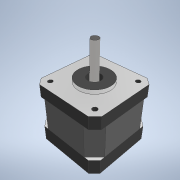
# Autodesk Inventor part: Nema-17
Saved by Autodesk Inventor 2021.1 (Build 251245010, 245A)
## iProperties
Created: 2022-01-16
Part Number: Nema-17
Material: Типовые
Document SubType Name: Modeling
Designer: Andrew
Density: 1 g/cm^3
Appearance: По умолчанию
Author: Andrew
Autodesk Inventor part; units mm, degrees
ref_plane "YZ Plane" through (0, 0, 0) normal (1, 0, 0) x (0, 1, 0)
ref_plane "XZ Plane" through (0, 0, 0) normal (0, 1, 0) x (-1, 0, 0)
ref_plane "XY Plane" through (0, 0, 0) normal (0, 0, 1) x (1, 0, 0)
sketch "Эскиз1" plane through (0, 0, 0) normal (0, 1, 0) x (-1, 0, 0)
  line L0 (9, 9) -> (-33, 9)
  line L1 (-33, 9) -> (-33, -33)
  line L2 (-33, -33) -> (9, -33)
  line L3 (9, -33) -> (9, 9)
  line L4 (9, -29) -> (5, -33)
  line L5 (9, 9) -> (-33, -33) construction
  line L6 (9, -33) -> (-33, 9) construction
  line L7 (5, 9) -> (9, 5)
  line L8 (-33, 5) -> (-29, 9)
  line L9 (-33, -29) -> (-29, -33)
  line L10 (13.5, -3.75) -> (9, -3.75)
  line L11 (9, -20.25) -> (13.5, -20.25)
  line L12 (13.5, -20.25) -> (13.5, -3.75)
  point P0 (0, 0)
  dimension "d0" = 42
  dimension "d1" = 42
  dimension "d2" = 4
  dimension "d3" = 4
  dimension "d17" = 12.75
  dimension "d18" = 16.5
  dimension "d19" = 4.5
  constraints: 26 end point, 10 point on line, 6 perpendicular, 2 parallel, 1 horizontal
  measures "d0" distance of L2.end L1.end
  measures "d1" distance of L1.end L0.end
  measures "d2" distance of L2.end L4.start
  measures "d3" distance of L4.end L2.end
  measures "d17" distance between parallel lines of L0 L10
  measures "d18" distance of L11.end L10.start
  measures "d19" distance of L11.start L11.end
extrude "Выдавливание1" add sketch "Эскиз1" along normal blind 9.5 contours L7 L3 L4 L2 L9 L1 L8 L0 | L10 L12 L11 L3
sketch "Эскиз2" plane through (0, 0, 0) normal (0, -1, 0) x (1, 0, 0)
  line L0 (-9, -33) -> (33, -33)
  line L1 (33, -33) -> (33, 9)
  line L2 (33, 9) -> (-9, 9)
  line L3 (-9, 9) -> (-9, -33)
  line L4 (-9, -33) -> (33, 9) construction
  line L5 (33, -33) -> (-9, 9) construction
  circle A0 centre (12, -12) radius 4.5
  circle A1 centre (-3.5, -27.5) radius 3.25
  circle A2 centre (-3.5, 3.5) radius 3.25
  circle A3 centre (27.5, 3.5) radius 3.25
  circle A4 centre (27.5, -27.5) radius 3.25
  line L6 (33, 5) -> (33, -29) projected
  line L7 (-5, 9) -> (29, 9) projected
  line L8 (29, -33) -> (-5, -33) projected
  line L9 (-9, -3.75) -> (-9, 5) projected
  point P0 (0, 0)
  dimension "d22" = 9
  dimension "d23" = 6.5
  dimension "d25" = 5.5
  dimension "d28" = 360
  constraints: 12 end point, 5 centre point, 4 collinear, 3 coincident, 2 parallel, 1 horizontal, 1 midpoint, 1 perpendicular, 1 point on line, 11 other
  measures "d22" diameter of A0
  measures "d23" diameter of A1
  measures "d25" distance from line of L0 A1.centre
extrude "Выдавливание2" cut sketch "Эскиз2" against normal blind 5 contours A0 | A1 | A2 | A3 | A4
sketch "Эскиз3" plane through (0, 9.5, 0) normal (0, 1, 0) x (1, 0, 0)
  line L0 (-13.5, 3.75) -> (-9, 3.75) projected
  line L1 (-13.5, 3.75) -> (-9, 3.75)
  line L2 (-9, 3.75) -> (-9, 20.25)
  line L3 (-9, 20.25) -> (-13.5, 20.25)
  line L4 (-13.5, 20.25) -> (-13.5, 3.75)
  point P0 (0, 0)
  constraints: 8 end point, 2 parallel, 1 horizontal, 1 perpendicular
extrude "Выдавливание3" cut sketch "Эскиз3" against normal blind 6
sketch "Эскиз4" plane through (-9, 0, -29) normal (-1, 0, 0) x (0, 0, 1)
  line L0 (8.75, 3.5) -> (25.25, 3.5) projected
  line L1 (8.75, 3.5) -> (25.25, 3.5)
  line L2 (25.25, 3.5) -> (25.25, 9.5)
  line L3 (25.25, 9.5) -> (8.75, 9.5)
  line L4 (8.75, 9.5) -> (8.75, 3.5)
  point P0 (29, 0)
  dimension "d34" = 16.5
  dimension "d35" = 6
  constraints: 8 end point, 2 parallel, 1 horizontal, 1 perpendicular
  measures "d34" distance of L3.end L2.end
  measures "d35" distance of L2.end L1.end
extrude "Выдавливание4" add sketch "Эскиз4" along normal blind 6 separate body
sketch "Эскиз5" plane through (-15, 0, -29) normal (-1, 0, 0) x (0, 0, 1)
  line L0 (25.25, 9.5) -> (8.75, 9.5) projected
  line L1 (25.25, 3.5) -> (8.75, 3.5) projected
  line L2 (8.75, 9.5) -> (25.25, 9.5)
  line L3 (25.25, 9.5) -> (25.25, 3.5)
  line L4 (25.25, 3.5) -> (8.75, 3.5)
  line L5 (8.75, 3.5) -> (8.75, 9.5)
  line L6 (9.75, 8.5) -> (12.75, 8.5)
  line L7 (24.25, 8.5) -> (24.25, 4.5)
  line L8 (24.25, 4.5) -> (9.75, 4.5)
  line L9 (9.75, 4.5) -> (9.75, 8.5)
  line L10 (12.75, 8.5) -> (12.75, 9.5)
  line L11 (21.25, 8.5) -> (21.25, 9.5)
  line L12 (0, 9.5) -> (34, 9.5) projected
  line L13 (21.25, 8.5) -> (24.25, 8.5)
  point P0 (29, 0)
  dimension "d38" = 1
  dimension "d39" = 4
  dimension "d40" = 4
  constraints: 22 end point, 5 parallel, 5 perpendicular, 3 point on line, 1 horizontal, 2 other
  measures "d38" distance between parallel lines of L5 L9
  measures "d39" distance between parallel lines of L10 L5
  measures "d40" distance between parallel lines of L11 L3
extrude "Выдавливание5" cut sketch "Эскиз5" against normal blind 6 contours L11 L13 L7 L8 L9 L6 L10 L0 bodies 2
sketch "Эскиз6" plane through (-9, 0, -29) normal (-1, 0, 0) x (0, 0, 1)
  line L0 (11.75, 7) -> (12.25, 7)
  line L1 (12.25, 7) -> (12.25, 6.5)
  line L2 (12.25, 6.5) -> (11.75, 6.5)
  line L3 (11.75, 6.5) -> (11.75, 7)
  line L4 (13.75, 7) -> (14.25, 7)
  line L5 (14.25, 7) -> (14.25, 6.5)
  line L6 (14.25, 6.5) -> (13.75, 6.5)
  line L7 (13.75, 6.5) -> (13.75, 7)
  line L8 (15.75, 7) -> (16.25, 7)
  line L9 (16.25, 7) -> (16.25, 6.5)
  line L10 (16.25, 6.5) -> (15.75, 6.5)
  line L11 (15.75, 6.5) -> (15.75, 7)
  line L12 (17.75, 7) -> (18.25, 7)
  line L13 (18.25, 7) -> (18.25, 6.5)
  line L14 (18.25, 6.5) -> (17.75, 6.5)
  line L15 (17.75, 6.5) -> (17.75, 7)
  line L16 (19.75, 7) -> (20.25, 7)
  line L17 (20.25, 7) -> (20.25, 6.5)
  line L18 (20.25, 6.5) -> (19.75, 6.5)
  line L19 (19.75, 6.5) -> (19.75, 7)
  line L20 (21.75, 7) -> (22.25, 7)
  line L21 (22.25, 7) -> (22.25, 6.5)
  line L22 (22.25, 6.5) -> (21.75, 6.5)
  line L23 (21.75, 6.5) -> (21.75, 7)
  line L24 (8.75, 0) -> (8.75, 3.5) projected
  point P0 (29, 0)
  dimension "d43" = 0.5
  dimension "d44" = 0.5
  dimension "d47" = 2
  dimension "d52" = 3
  constraints: 48 end point, 2 horizontal, 2 parallel, 1 collinear, 1 perpendicular, 39 other
  measures "d43" distance of L1.end L2.end
  measures "d44" distance of L0.end L1.end
  measures "d47" distance of L0.start L4.start
  measures "d52" distance between parallel lines of L24 L3
extrude "Выдавливание6" add sketch "Эскиз6" along normal blind 5 separate body
sketch "Эскиз7" plane through (0, 9.5, 0) normal (0, 1, 0) x (1, 0, 0)
  line L0 (33, 33) -> (-9, 33)
  line L1 (-9, 33) -> (-9, -9)
  line L2 (-9, -9) -> (33, -9)
  line L3 (33, -9) -> (33, 33)
  line L4 (33, -2) -> (26, -9)
  line L5 (33, -5) -> (33, 29) projected
  line L6 (-5, -9) -> (29, -9) projected
  line L7 (-9, 29) -> (-9, -5) projected
  line L8 (-9, -2) -> (-2, -9)
  line L9 (-2, 33) -> (-9, 26)
  line L10 (33, 26) -> (26, 33)
  line L11 (29, 33) -> (-5, 33) projected
  point P0 (0, 0)
  point P1 (33, 12)
  point P2 (12, -9)
  point P3 (-2, -9)
  dimension "d56" = 7
  dimension "d57" = 42
  dimension "d58" = 42
  dimension "d59" = 7
  constraints: 16 end point, 7 point on line, 4 midpoint, 2 parallel, 2 perpendicular, 1 horizontal
  measures "d56" distance from line of L4.start L2
  measures "d57" distance of L2.end L0.start
  measures "d58" distance of L1.end L2.end
  measures "d59" distance from line of L3 L4.end
extrude "Выдавливание7" add sketch "Эскиз7" along normal blind 20 separate body contours L10 L3 L4 L2 L8 L1 L9 L0
sketch "Эскиз8" plane through (0, 29.5, 0) normal (0, 1, 0) x (1, 0, 0)
  line L0 (33, 33) -> (-9, 33)
  line L1 (-9, 33) -> (-9, -9)
  line L2 (-9, -9) -> (33, -9)
  line L3 (33, -9) -> (33, 33)
  line L4 (33, 29) -> (29, 33)
  line L5 (29, -9) -> (33, -5)
  line L6 (-9, -5) -> (-5, -9)
  line L7 (-9, 29) -> (-5, 33)
  point P0 (0, 0)
  dimension "d62" = 42
  dimension "d63" = 42
  dimension "d64" = 4
  dimension "d65" = 4
  constraints: 16 end point, 8 point on line, 3 perpendicular, 2 parallel, 1 horizontal
  measures "d62" distance of L2.end L1.end
  measures "d63" distance of L1.end L0.end
  measures "d64" distance from line of L0 L4.start
  measures "d65" distance from line of L3 L4.end
extrude "Выдавливание8" add sketch "Эскиз8" along normal blind 7.6 contours L4 L3 L5 L2 L6 L1 L7 L0 bodies 1
sketch "Эскиз9" plane through (0, 37.1, 0) normal (0, 1, 0) x (1, 0, 0)
  line L0 (33, -9) -> (-9, -9)
  line L1 (-9, -9) -> (-9, 33)
  line L2 (-9, 33) -> (33, 33)
  line L3 (33, 33) -> (33, -9)
  line L4 (33, -9) -> (-9, 33) construction
  line L5 (-9, -9) -> (33, 33) construction
  circle A0 centre (12, 12) radius 11
  point P0 (0, 0)
  dimension "d68" = 42
  dimension "d69" = 42
  dimension "d70" = 22
  constraints: 12 end point, 2 parallel, 1 centre point, 1 horizontal, 1 midpoint, 1 perpendicular
  measures "d68" distance of L1.end L2.end
  measures "d69" distance of L0.end L1.end
  measures "d70" diameter of A0
extrude "Выдавливание9" add sketch "Эскиз9" along normal blind 2.5 contours A0 bodies 1
sketch "Эскиз10" plane through (12, 39.6, -12) normal (0, 1, 0) x (1, 0, 0)
  circle A0 centre (0, 0) radius 11 projected
  circle A1 centre (0, 0) radius 4.5
  point P0 (-12, -12)
  dimension "d73" = 9
  constraints: 1 centre point, 1 coincident
  measures "d73" diameter of A1
extrude "Выдавливание10" cut sketch "Эскиз10" against normal blind 5 contours A1 bodies 1
sketch "Эскиз11" plane through (12, 34.6, -12) normal (0, 1, 0) x (1, 0, 0)
  circle A0 centre (0, 0) radius 4.5 projected
  circle A1 centre (0, 0) radius 2.5
  point P0 (-12, -12)
  dimension "d76" = 5
  constraints: 1 centre point, 1 coincident
  measures "d76" diameter of A1
extrude "Выдавливание11" add sketch "Эскиз11" along normal blind 26 contours A1 bodies 1
sketch "Эскиз12" plane through (12, 60.6, -12) normal (0, 1, 0) x (1, 0, 0)
  circle A0 centre (0, 0) radius 2.5 projected
  line L0 (-2.5, 0) -> (-0.6992, -2.4002)
  circle A1 centre (0, 0) radius 2.5
  point P0 (-12, -12)
  constraints: 2 end point, 2 point on circle, 1 centre point, 1 coincident, 1 concentric
extrude "Выдавливание12" cut sketch "Эскиз12" against normal blind 18 contours L0 A0 picked at (-1.8806, -0.9775) bodies 1
sketch "Эскиз13" plane through (0, 37.1, 0) normal (0, 1, 0) x (1, 0, 0)
  line L0 (-9, -9) -> (33, -9)
  line L1 (33, -9) -> (33, 33)
  line L2 (33, 33) -> (-9, 33)
  line L3 (-9, 33) -> (-9, -9)
  circle A0 centre (27.5, 27.5) radius 1.5
  circle A1 centre (-3.5, -3.5) radius 1.5
  line L4 (-9, 29) -> (-9, -5) projected
  line L5 (-9, 27.5) -> (33, 27.5) construction
  line L6 (33, -5) -> (33, 29) projected
  line L7 (29, 33) -> (-5, 33) projected
  line L8 (27.5, 33) -> (27.5, -9) construction
  line L9 (-5, -9) -> (29, -9) projected
  line L10 (-9, -3.5) -> (33, -3.5) construction
  line L11 (33, -5) -> (33, 29) projected
  line L12 (-3.5, -9) -> (-3.5, 33) construction
  line L13 (29, 33) -> (-5, 33) projected
  circle A2 centre (-3.5, 27.5) radius 1.5
  circle A3 centre (27.5, -3.5) radius 1.5
  point P0 (0, 0)
  dimension "d81" = 42
  dimension "d82" = 42
  dimension "d85" = 3
  dimension "d86" = 3
  dimension "d89" = 5.5
  dimension "d90" = 5.5
  dimension "d91" = 5.5
  dimension "d92" = 5.5
  dimension "d93" = 3
  dimension "d94" = 3
  constraints: 16 end point, 16 point on line, 5 perpendicular, 4 centre point, 2 parallel, 1 horizontal
  measures "d81" distance of L2.end L1.end
  measures "d82" distance of L1.end L0.end
  measures "d85" diameter of A0
  measures "d86" diameter of A1
  measures "d89" distance between parallel lines of L7 L5
  measures "d90" distance between parallel lines of L3 L12
  measures "d91" distance between parallel lines of L1 L8
  measures "d92" distance between parallel lines of L0 L10
  measures "d93" diameter of A2
  measures "d94" diameter of A3
extrude "Выдавливание13" cut sketch "Эскиз13" against normal blind 5 contours A0 | A1 | A2 | A3 bodies 1
equation "\"d85\" = d93"
equation "\"d86\" = d93"
equation "\"d90\" = d89"
equation "\"d91\" = d89"
equation "\"d92\" = d89"
equation "\"d94\" = d93"
